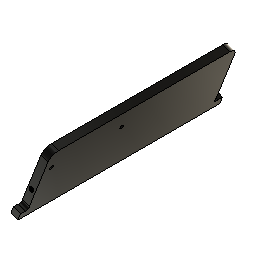
CameraHolderNew v3 (Autodesk Fusion 360 design; units mm, degrees)
Autodesk Fusion 360 part; units mm, degrees
ref_plane "WorkPlane1" through (0, 12.125, 0) normal (0.932008, 0, -0.362438) x (0, 1, 0)
sketch "Sketch1" plane through (0, 12.125, 0) normal (0.932008, 0, -0.362438) x (0, 1, 0)
  line L0 (-55, 22.5) -> (55, 22.5)
  line L1 (60, -22.5) -> (-60, -22.5)
  line L2 (-60, 22.5) -> (60, -22.5) construction
  line L3 (-60, -22.5) -> (-65, -22.5)
  line L4 (-65, -22.5) -> (-65, -17.7)
  line L5 (-65, -17.7) -> (-62.1213, -17.7)
  line L6 (-60, -17.7) -> (-61.0607, -16.6393) construction
  arc A0 (-62.1213, -17.7) -> (-60, -15.5787) centre (-61.0607, -16.6393) ccw
  arc A1 (-60, -15.5787) -> (-62.1213, -17.7) centre (-61.0607, -16.6393) ccw construction
  line L7 (-62.1213, -17.7) -> (-60, -17.7) construction
  line L8 (-60, -22.5) -> (-60, -17.7) construction
  line L9 (-60, -15.5787) -> (-60, 17.5)
  line L10 (-60, -17.7) -> (-60, -15.5787) construction
  circle A2 centre (-55, 10) radius 1.25
  circle A3 centre (-10, 10) radius 1.25
  line L11 (0, 0) -> (0, 10) construction
  line L12 (0, 10) -> (-60, 10) construction
  line L13 (60, -22.5) -> (65, -22.5)
  line L14 (65, -22.5) -> (65, -17.7)
  line L15 (65, -17.7) -> (62.1213, -17.7)
  line L16 (60, -17.7) -> (61.0607, -16.6393) construction
  arc A4 (60, -15.5787) -> (62.1213, -17.7) centre (61.0607, -16.6393) ccw
  arc A5 (62.1213, -17.7) -> (60, -15.5787) centre (61.0607, -16.6393) ccw construction
  line L17 (62.1213, -17.7) -> (60, -17.7) construction
  line L18 (60, 17.5) -> (60, -15.5787)
  line L19 (60, -17.7) -> (60, -22.5) construction
  line L20 (60, -15.5787) -> (60, -17.7) construction
  arc A6 (-55, 22.5) -> (-60, 17.5) centre (-55, 17.5) ccw
  arc A7 (60, 17.5) -> (55, 22.5) centre (55, 17.5) ccw
  line L21 (-60, -2.5) -> (0, -2.5) construction
  line L22 (0, -2.5) -> (0, 0) construction
  line L23 (-60, -5.7) -> (60, -5.7) construction
  line L24 (-60, -4.2) -> (-52, -4.2) construction
  line L25 (-52, -4.2) -> (-52, -7.2) construction
  line L26 (-52, -7.2) -> (-60, -7.2) construction
  line L27 (60, -4.2) -> (52, -4.2) construction
  line L28 (52, -4.2) -> (52, -7.2) construction
  line L29 (52, -7.2) -> (60, -7.2) construction
  point P0 (60, 22.5)
  point P1 (-52, -5.7)
  point P2 (52, -5.7)
  dimension "d3" = 120
  dimension "d4" = 5
  dimension "d5" = 4.8
  dimension "d6" = 1.5
  dimension "d7" = 45
  dimension "d9" = 2.5
  dimension "d10" = 2.5
  dimension "d12" = 45
  dimension "d13" = 10
  dimension "d15" = 12.5
  dimension "d16" = 5
  dimension "d17" = 4.8
  dimension "d18" = 1.5
  dimension "d19" = 45
  dimension "d20" = 5
  dimension "d21" = 5
  dimension "d22" = 25
  dimension "d23" = 45
  dimension "d24" = 12
  dimension "d25" = 3
  dimension "d26" = 8
  dimension "d27" = 3
  dimension "d28" = 8
  constraint horizontal L0
  constraint vertical L18
  constraint horizontal L1
  constraint vertical L8
  constraint coincident L11.start L22.end
  constraint perpendicular L3 L8
  constraint perpendicular L3 L4
  constraint perpendicular L5 L8
  constraint coincident L6.end A0.centre
  constraint coincident L6.start A0
  constraint coincident A0.end L8
  constraint concentric A0 A1
  constraint perpendicular L7 L8
  constraint collinear L9 L10
  constraint coincident L9 L12.end
  constraint perpendicular L9 L12
  constraint coincident A2.centre L12
  constraint coincident A3.centre L12
  constraint perpendicular L11 L12
  constraint perpendicular L13 L18
  constraint perpendicular L13 L14
  constraint coincident L16.start L18
  constraint perpendicular L15 L18
  constraint coincident L16.end A4.centre
  constraint coincident L16.start A4
  constraint concentric A4 A5
  constraint perpendicular L17 L18
  constraint collinear L19 L20
  constraint coincident L2.start L9
  constraint coincident L2.start L0
  constraint tangent L9 A6
  constraint tangent L0 A6
  constraint coincident P0 L0
  constraint coincident P0 L18
  constraint tangent L0 A7
  constraint tangent L18 A7
  constraint coincident L9 L21.start
  constraint perpendicular L9 L21
  constraint perpendicular L21 L22
  constraint coincident L9 L23.start
  constraint coincident L18 L23.end
  constraint perpendicular L18 L23
  constraint coincident L9 L24.start
  constraint perpendicular L9 L24
  constraint perpendicular L24 L25
  constraint coincident L9 L26.end
  constraint perpendicular L9 L26
  constraint midpoint L25 P1
  constraint coincident L23 P1
  constraint coincident L18 L27.start
  constraint perpendicular L18 L27
  constraint perpendicular L23 L28
  constraint coincident L18 L29.end
  constraint perpendicular L18 L29
  constraint midpoint L28 P2
  constraint coincident L23 P2
  constraint midpoint L2 L11.start
  measures "d3" distance of L2.start P0
  measures "d4" distance of L1.end L3.end L1.start
  measures "d5" distance of L3.end L4.end
  measures "d6" distance of L6.start L6.end L1.start
  measures "d7" angle of L5 L6
  measures "d9" diameter of A2
  measures "d10" diameter of A3
  measures "d12" distance of A2.centre A3.centre
  measures "d13" horizontal distance of L11.start A3.centre
  measures "d15" distance of L0 L12
  measures "d16" distance of L1.start L13.end
  measures "d17" distance of L13.end L14.end
  measures "d18" distance of L16.start L16.end
  measures "d19" angle of L15 L16
  measures "d20" radius of A6
  measures "d21" radius of A7
  measures "d22" distance of L0 L21
  measures "d23" distance of L0 L1
  measures "d24" distance of L5 L23
  measures "d25" distance of L24.end L25.end
  measures "d26" distance of L25.end L26.end
  measures "d27" distance of L27.end L28.end
  measures "d28" distance of L28.end L29.end
extrude "Extrude1" add sketch "Sketch1" along normal blind 4.8
sketch "Sketch2" plane through (0, -47.875, 0) normal (0, -1, 0) x (1, 0, 0)
  line L0 (6.3427, 16.3101) -> (-5.6463, -14.5195)
  line L1 (-5.6463, -14.5195) -> (-1.1727, -16.2592)
  line L2 (-1.1727, -16.2592) -> (10.8163, 14.5704)
  line L3 (10.8163, 14.5704) -> (6.3427, 16.3101)
  line L4 (-2.0659, -5.3124) -> (0.1709, -6.1823) construction
  line L5 (-5.6463, -14.5195) -> (6.3427, 16.3101) construction
  circle A0 centre (0.1709, -6.1823) radius 1.5
  point P0 (-2.0659, -5.3124)
  dimension "d31" = 2.4
  dimension "d32" = 3
  constraint coincident P0 L4.start
  constraint perpendicular L0 L4
  constraint coincident L4.end A0.centre
  measures "d31" distance of P0 L4.end
  measures "d32" diameter of A0
sketch "Sketch3" plane through (0, 72.125, 0) normal (0, 1, 0) x (-1, 0, 0)
  line L0 (5.6463, -14.5195) -> (-6.3427, 16.3101)
  line L1 (-6.3427, 16.3101) -> (-10.8163, 14.5704)
  line L2 (-10.8163, 14.5704) -> (1.1727, -16.2592)
  line L3 (1.1727, -16.2592) -> (5.6463, -14.5195)
  line L4 (-6.3427, 16.3101) -> (5.6463, -14.5195)
  line L5 (2.0659, -5.3124) -> (-0.1709, -6.1823) construction
  circle A0 centre (-0.1709, -6.1823) radius 1.5
  point P0 (2.0659, -5.3124)
  dimension "d33" = 2.4
  dimension "d34" = 3
  constraint coincident P0 L5.start
  constraint perpendicular L4 L5
  constraint coincident L5.end A0.centre
  measures "d33" distance of P0 L5.end
  measures "d34" diameter of A0
extrude "Extrude2" cut sketch "Sketch2" against normal blind 8 contours A0
extrude "Extrude3" cut sketch "Sketch3" against normal blind 8 contours A0
thread "Thread1" "ISO Metric profile 3.0 M3x0.5 6H" major diameter 3.086 minor diameter 2.529 pitch 0.5 angle 60 modelled right hand crest width 0.1368 on face at (1.6635, -45.2083, -6.3316) crest through (1.4354, -47.75, -6.1823)
thread "Thread2" "ISO Metric profile 3.0 M3x0.5 6H" major diameter 3.086 minor diameter 2.529 pitch 0.5 angle 60 modelled right hand crest width 0.1368 on face at (-1.3272, 66.7917, -6.2571) crest through (-1.0936, 72, -6.1823)
